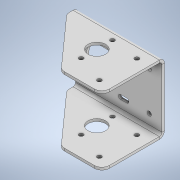
# Autodesk Inventor part: Z Drive Mount
Saved by Autodesk Inventor 2022 (Build 260153000, 153)
## iProperties
Created: 2021-10-05
Part Number: Z Drive Mount
Material: Generic
Document SubType Name: Sheet Metal
Designer: Administrator
Density: 1 g/cm^3
Appearance: Default
Sheet Metal Rule: 0.08in
Title: Z Drive Mount v7
Author: Administrator
Autodesk Inventor part; units mm, degrees
ref_plane "YZ Plane" through (0, 0, 0) normal (1, 0, 0) x (0, 1, 0)
ref_plane "XZ Plane" through (0, 0, 0) normal (0, 1, 0) x (-1, 0, 0)
ref_plane "XY Plane" through (0, 0, 0) normal (0, 0, 1) x (1, 0, 0)
sketch "Sketch1" plane through (0, 0, 0) normal (0, 0, 1) x (1, 0, 0)
  line L0 (0, 0) -> (69, 0)
  line L1 (69, 0) -> (69, 55)
  line L2 (69, 55) -> (0, 55)
  line L3 (0, 55) -> (0, 0)
  line L4 (38.5, 43) -> (38.5, 55) construction
  line L5 (38.5, 12) -> (38.5, 0) construction
  line L6 (69, 55) -> (49, 55) construction
  line L7 (49, 55) -> (49, 0) construction
  line L8 (49, 0) -> (69, 0) construction
  line L9 (69, 0) -> (69, 55) construction
  line L10 (49, 12) -> (69, 12) construction
  line L11 (5, 43) -> (10, 43) construction
  line L12 (5, 44.7) -> (10, 44.7)
  line L13 (10, 41.3) -> (5, 41.3)
  arc A0 (5, 44.7) -> (5, 41.3) centre (5, 43) ccw
  arc A1 (10, 41.3) -> (10, 44.7) centre (10, 43) ccw
  line L14 (36, 43) -> (41, 43) construction
  line L15 (36, 41.3) -> (41, 41.3)
  line L16 (41, 44.7) -> (36, 44.7)
  arc A2 (36, 44.7) -> (36, 41.3) centre (36, 43) ccw
  arc A3 (41, 41.3) -> (41, 44.7) centre (41, 43) ccw
  line L17 (5, 12) -> (10, 12) construction
  line L18 (5, 10.3) -> (10, 10.3)
  line L19 (10, 13.7) -> (5, 13.7)
  arc A4 (5, 13.7) -> (5, 10.3) centre (5, 12) ccw
  arc A5 (10, 10.3) -> (10, 13.7) centre (10, 12) ccw
  line L20 (36, 12) -> (41, 12) construction
  line L21 (36, 13.7) -> (41, 13.7)
  line L22 (41, 10.3) -> (36, 10.3)
  arc A6 (36, 13.7) -> (36, 10.3) centre (36, 12) ccw
  arc A7 (41, 10.3) -> (41, 13.7) centre (41, 12) ccw
  line L23 (20.5, 27.5) -> (25.5, 27.5) construction
  line L24 (20.5, 39.5) -> (25.5, 39.5)
  line L25 (25.5, 15.5) -> (20.5, 15.5)
  arc A8 (20.5, 39.5) -> (20.5, 15.5) centre (20.5, 27.5) ccw
  arc A9 (25.5, 15.5) -> (25.5, 39.5) centre (25.5, 27.5) ccw
  line L26 (38.5, 43) -> (7.5, 12) construction
  point P0 (59, 43)
  point P1 (59, 12)
  point P2 (59, 12)
  point P3 (7.5, 43)
  point P4 (23, 27.5)
  point P5 (23, 27.5)
  dimension "d1" = 55
  dimension "d2" = 20
  dimension "d8" = 31
  dimension "d9" = 31
  dimension "d10" = 31
  dimension "d11" = 1.7
  dimension "d12" = 5
  dimension "d13" = 12
  dimension "d14" = 5
  dimension "d15" = 5
  dimension "d53" = 69
  constraints: 64 end point, 20 point on circle, 20 tangent, 10 centre point, 10 parallel, 7 midpoint, 6 point on line, 5 horizontal, 5 perpendicular, 4 coincident, 4 equal length, 3 equal radius, 2 collinear, 2 horizontal alignment, 2 vertical alignment, 1 vertical
  measures "d1" distance of L0.start L2.end
  measures "d2" distance of L8.end L7.end
  measures "d8" distance of L26.end point (38.5, 12)
  measures "d9" distance of L26.start point (38.5, 12)
  measures "d10" distance of point (7.5, 43) L26.start
  measures "d11" radius of A3
  measures "d12" distance of L14.start L14.end
  measures "d13" radius of A8
  measures "d14" distance of L23.start L23.end
  measures "d15" distance from line of L3 L11.start
  measures "d53" distance between parallel lines of L1 L3
extrude "Plate1" add sketch "Sketch1" along normal blind 2.032
hole "Hole1" at (59, 12, 0) at (59, 43, 0) direction (0, 0, 1) diameter 3.4 depth 2.032 tip angle 118 clearance for "Socket Head Cap Screw" size "M3" standard "Ansi Metric M Profile"
sketch "Sketch2" plane through (0, 52.968, 0) normal (0, 1, 0) x (-1, 0, 0)
  line L0 (-69, 0) -> (0, 0)
  line L1 (0, 0) -> (0, 50)
  line L2 (0, 50) -> (-69, 50)
  line L3 (-69, 50) -> (-69, 0)
  constraints: 6 end point, 1 horizontal, 1 perpendicular, 1 vertical
edge flange "Flange1" height 50 angle 90 thickness 2.032 bend radius 2.032 thickness toward (0, 1, 0) relief straight relief width 2.032 relief depth 1.016 corner gap 2.032 corner form 0 edges at (34.5, 55, 2.032) (34.5, 0, 2.032) wall of the first edge with corners at (69, 52.968, 0) (0, 52.968, 0) (0, 52.968, 50) (69, 52.968, 50)
bend "Bend1"
corner "Corner1"
sketch "Sketch3" plane through (0, 0, 50) normal (0, -1, 0) x (1, 0, 0)
  line L0 (69, -45.936) -> (69, 0) construction
  line L1 (69, 0) -> (49, 0) construction
  line L2 (49, 0) -> (49, -45.936) construction
  line L3 (49, -45.936) -> (69, -45.936) construction
  line L4 (69, -45.936) -> (69, 0) construction
  line L5 (49, -37.968) -> (69, -37.968) construction
  line L6 (59, -7.968) -> (59, 0) construction
  line L7 (69, 0) -> (0, 0) construction
  line L8 (59, -37.968) -> (59, -45.936) construction
  line L9 (69, -45.936) -> (0, -45.936) construction
  circle A0 centre (36.5, -28.436) radius 7
  line L10 (0, -45.936) -> (0, 0) projected
  line L11 (0, -40.936) -> (36.5, 0)
  line L12 (0, 0) -> (69, 0) projected
  point P0 (0, -50)
  point P1 (36.5, -15.936)
  point P2 (36.5, -40.936)
  dimension "d34" = 20
  dimension "d35" = 30
  dimension "d36" = 14
  dimension "d37" = 12.5
  dimension "d38" = 12.5
  dimension "d39" = 5
  dimension "d40" = 12.5
  constraints: 16 end point, 6 point on line, 4 perpendicular, 4 vertical alignment, 2 parallel, 1 centre point, 1 coincident, 1 collinear, 1 horizontal, 1 horizontal alignment, 1 midpoint
  measures "d34" distance of L3.end L2.end
  measures "d35" distance of L6.start L8.start
  measures "d36" diameter of A0
  measures "d37" distance of point (36.5, -15.936) A0.centre
  measures "d38" distance of point (36.5, -40.936) A0.centre
  measures "d39" distance from line of point (36.5, -40.936) L9
  measures "d40" distance from line of L2 A0.centre
extrude "Cut1" cut sketch "Sketch3" against normal through all contours A0
hole "Hole2" at (36.5, 0, 34.064) at (36.5, 0, 9.064) at (59, 0, 42.032) at (59, 0, 12.032) direction (0, 1, 0) diameter 3.4 depth 55 tip angle 118 clearance for "Socket Head Cap Screw" size "M3" standard "Ansi Metric M Profile"
extrude "Cut2" cut sketch "Sketch3" against normal through all contours L10 L12 L11
fillet "Corner Round1" radius 6 6 edges at (0, 53.984, 9.064) (0, 1.016, 9.064) (36.5, 1.016, 50) (36.5, 53.984, 50) (69, 53.984, 50) (69, 1.016, 50)
equation "\"d8\" = d10"
equation "\"d9\" = d10"
equation "\"d22\" = Thickness"
equation "\"d41\" = Thickness"
equation "\"d50\" = Thickness"
equation "\"d16\" = Thickness"
equation "\"d24\" = BendReliefWidth"
equation "\"d25\" = BendReliefDepth"
equation "\"d26\" = MinimumRemnant"
equation "\"d27\" = TransitionRadius"
equation "\"d30\" = BendRadius"
equation "\"d31\" = CornerReliefSize"
equation "\"d32\" = GapSize"
equation "\"d33\" = JacobiRadiusSize"
equation "\"BendRadius\" = Thickness"
equation "\"BendReliefWidth\" = Thickness"
equation "\"BendReliefDepth\" = 0.5 * Thickness"
equation "\"CornerReliefSize\" = 4 * Thickness"
equation "\"MinimumRemnant\" = 2 * Thickness"
equation "\"TransitionRadius\" = BendRadius"
equation "\"JacobiRadiusSize\" = BendRadius"
equation "\"GapSize\" = Thickness"
equation "\"d7\" = d4"
equation "\"Thickness\" = 2.032"
equation "\"d4\" = 31"
body "Solid1"
body "Solid2"
